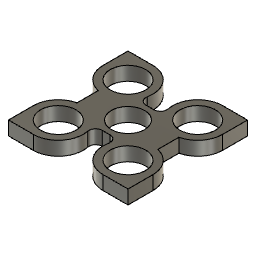
Model 23 (Autodesk Fusion 360 design; units mm, degrees)
Autodesk Fusion 360 part; units mm, degrees
note: some values were not read from the file. Set by a fixed rule: which sketch regions a step uses.
sketch "Sketch1" plane through (0, 0, 0) normal (0, 0, 1) x (1, 0, 0)
  circle A0 centre (0, 0) radius 30
  line L0 (0, 0) -> (0, 63) construction
  line L1 (0, 63) -> (63, 63) construction
  line L2 (0, 63) -> (-63, 63) construction
  circle A1 centre (-63, 63) radius 32
  circle A2 centre (63, 63) radius 32
  line L3 (0, 0) -> (0, -63) construction
  line L4 (0, -63) -> (-63, -63) construction
  line L5 (0, -63) -> (63, -63) construction
  circle A3 centre (-63, -63) radius 32
  circle A4 centre (63, -63) radius 32
  line L6 (-63, 108) -> (-108, 108)
  line L7 (-63, 63) -> (-108, 63) construction
  line L8 (-108, 63) -> (-108, 108)
  line L9 (63, 63) -> (108, 63) construction
  line L10 (108, 63) -> (108, 108)
  line L11 (63, 63) -> (63, 108) construction
  line L12 (63, 108) -> (108, 108)
  line L13 (63, -63) -> (63, -108) construction
  line L14 (63, -108) -> (108, -108)
  line L15 (63, -63) -> (108, -63) construction
  line L16 (108, -63) -> (108, -108)
  line L17 (-63, -63) -> (-108, -63) construction
  line L18 (-108, -63) -> (-108, -108)
  line L19 (-63, -63) -> (-63, -108) construction
  line L20 (-63, -108) -> (-108, -108)
  line L21 (0, 0) -> (73, 0) construction
  line L22 (0, 0) -> (-73, 0) construction
  line L23 (-73, -19.1252) -> (-73, 19.1252)
  line L24 (73, 0) -> (73, 19.1252)
  line L25 (73, 0) -> (73, -19.1252)
  arc A5 (7.1703, 39.5031) -> (18.9249, 53.9235) centre (7.1715, 51.5031) ccw
  arc A6 (-7.1674, -39.5031) -> (-18.9249, -53.9235) centre (-7.1715, -51.5031) ccw
  arc A7 (18.9249, -53.9235) -> (6.8327, -39.5079) centre (7.1715, -51.5031) ccw
  line L26 (-5.6873, 39.5952) -> (-5.6767, 39.5952)
  line L27 (6.8327, -39.5079) -> (-7.1674, -39.5031)
  arc A8 (-63, -108) -> (-18.9249, -53.9235) centre (-63, -63) ccw
  arc A9 (-73, -19.1252) -> (-108, -63) centre (-63, -63) ccw
  arc A10 (108, -63) -> (73, -19.1252) centre (63, -63) ccw
  arc A11 (18.9249, -53.9235) -> (63, -108) centre (63, -63) ccw
  arc A12 (63, 108) -> (18.9249, 53.9235) centre (63, 63) ccw
  arc A13 (73, 19.1252) -> (108, 63) centre (63, 63) ccw
  arc A14 (-108, 63) -> (-73, 19.1252) centre (-63, 63) ccw
  arc A15 (-18.9249, 53.9235) -> (-63, 108) centre (-63, 63) ccw
  line L28 (7.1703, 39.5031) -> (-7.1715, 39.5031)
  arc A16 (-18.9249, 53.9235) -> (-6.9894, 39.5045) centre (-7.1715, 51.5031) ccw
  dimension "d1" = 60
  dimension "d3" = 63
  dimension "d4" = 63
  dimension "d5" = 63
  dimension "d6" = 64
  dimension "d7" = 90
  dimension "d8" = 64
  dimension "d9" = 90
  dimension "d10" = 63
  dimension "d11" = 63
  dimension "d12" = 63
  dimension "d13" = 64
  dimension "d14" = 90
  dimension "d15" = 64
  dimension "d16" = 90
  dimension "d17" = 73
  dimension "d18" = 73
  dimension "d21" = 24
  dimension "d22" = 24
  dimension "d24" = 38.2504
  constraint coincident A0.centre L0.start
  constraint vertical L0
  constraint perpendicular L0 L1
  constraint perpendicular L0 L2
  constraint coincident L2.end A1.centre
  constraint concentric A1 A14
  constraint coincident L1.end A2.centre
  constraint concentric A2 A12
  constraint parallel L0 L3
  constraint perpendicular L3 L4
  constraint perpendicular L3 L5
  constraint coincident L4.end A3.centre
  constraint concentric A3 A8
  constraint coincident L5.end A4.centre
  constraint concentric A4 A10
  constraint coincident L6.start A14
  constraint tangent L6 A14
  constraint parallel L2 L7
  constraint perpendicular L6 L8
  constraint parallel L1 L9
  constraint perpendicular L9 L10
  constraint perpendicular L9 L11
  constraint tangent L12 A12
  constraint perpendicular L5 L13
  constraint tangent L14 A10
  constraint parallel L5 L15
  constraint perpendicular L14 L16
  constraint horizontal L17
  constraint tangent L18 A8
  constraint perpendicular L4 L19
  constraint tangent L20 A8
  constraint coincident L6 A15.end
  constraint perpendicular L3 L21
  constraint perpendicular L0 L22
  constraint perpendicular L22 L23
  constraint coincident L23.start A8
  constraint coincident L24.end A12
  constraint perpendicular L21 L24
  constraint perpendicular L21 L25
  constraint coincident A15.start A14
  constraint tangent A6 A8
  constraint tangent A7 A10
  constraint coincident A7.start A10
  constraint tangent A5 L26
  constraint tangent A6 L27
  constraint concentric A8 A9
  constraint concentric A10 A11
  constraint concentric A12 A13
  constraint concentric A14 A15
  constraint coincident L28.end A16
  constraint tangent L28 A16
  measures "d1" diameter of A0
  measures "d3" distance of A0.centre L0.end
  measures "d4" distance of L0.end L1.end
  measures "d5" distance of L0.end L2.end
  measures "d6" diameter of A1
  measures "d7" diameter of A14
  measures "d8" diameter of A2
  measures "d9" diameter of A12
  measures "d10" distance of A0.centre L3.end
  measures "d11" distance of L3.end L4.end
  measures "d12" distance of L3.end L5.end
  measures "d13" diameter of A3
  measures "d14" diameter of A8
  measures "d15" diameter of A4
  measures "d16" diameter of A10
  measures "d17" distance of A0.centre L21.end
  measures "d18" distance of A0.centre L22.end
  measures "d21" diameter of A6
  measures "d22" diameter of A7
  measures "d24" distance of L23.end L23.start
extrude "Extrude1" add sketch "Sketch1" along normal blind 25
